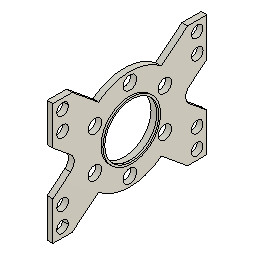
Ru28_Connector (Autodesk Fusion 360 design; units mm, degrees)
Autodesk Fusion 360 part; units mm, degrees
sketch "Sketch1" plane through (0, 0, 0) normal (0, 0, 1) x (1, 0, 0) in component "FINALBASE__2.0 v63"
  line L0 (175, -25) -> (0, -25)
  line L1 (0, -25) -> (0, 25)
  line L2 (0, 25) -> (175, 25)
  line L3 (175, 25) -> (175, -25)
  constraint horizontal L0
  constraint vertical L1
  constraint horizontal L2
  constraint vertical L3
extrude "Extrude1" add sketch "Sketch1" along normal blind 5 makes body 1 in component "FINALBASE__2.0 v63"
sketch "Sketch2" plane through (175, 0, 0) normal (1, 0, 0) x (0, 1, 0) in component "FINALBASE__2.0 v63"
  circle A0 centre (-0.0248, 31.4535) radius 20.9965 construction
  circle A1 centre (-0.0248, 31.4535) radius 22.3327
  line L0 (25, 0) -> (-25.0497, 0)
  line L1 (-25.0497, 0) -> (-25.0497, 62.9071)
  line L2 (-25.0497, 62.9071) -> (25, 62.9071)
  line L3 (25, 62.9071) -> (25, 0)
  line L4 (25, 0) -> (-25.0497, 62.9071) construction
  line L5 (-25.0497, 0) -> (25, 62.9071) construction
  line L6 (-0.0248, 31.4535) -> (-25.0497, 31.4535)
  line L7 (-0.0248, 31.4535) -> (25, 31.4535)
  point P0 (-0.0248, 31.4535)
  constraint concentric A0 A1
  constraint horizontal L0
  constraint perpendicular L0 L1
  constraint parallel L0 L2
  constraint parallel L1 L3
  constraint coincident L4 P0
  constraint coincident L5 P0
  constraint coincident P0 A0.centre
  constraint midpoint L1 L6.end
  constraint midpoint L3 L7.end
extrude "Extrude2" add sketch "Sketch2" along normal blind -52 and the other way blind 14 contours A1 L0 L1 L3 L6 L7 bodies 1 in component "FINALBASE__2.0 v63"
extrude "Extrude3" add 1 faces at (123, 0.548, 6.3944) along direction (-1, 0, 0) blind 95 and the other way blind -42 on bodies 1 bodies 1 in component "FINALBASE__2.0 v63"
fillet "Fillet1" radius 5 2 edges at (81, 0, 5) (123, 0, 5) on bodies 1 in component "FINALBASE__2.0 v63"
sketch "Sketch3" plane through (0, 0, 31.4535) normal (0, 0, 1) x (-1, 0, 0) in component "FINALBASE__2.0 v63"
  line L0 (-161, -25) -> (-123, -25) construction
  line L1 (-123, -25) -> (-123, 25) construction
  line L2 (-123, 25) -> (-161, 25) construction
  line L3 (-161, 25) -> (-161, -25) construction
  line L4 (-81, -25) -> (-28, -25) construction
  line L5 (-28, -25) -> (-28, 25) construction
  line L6 (-28, 25) -> (-81, 25) construction
  line L7 (-81, 25) -> (-81, -25) construction
  line L8 (-161, 25) -> (-123, 25)
  line L9 (-123, 25) -> (-123, 40)
  line L10 (-123, 40) -> (-161, 40)
  line L11 (-161, 40) -> (-161, 25)
  line L12 (-161, -25) -> (-123, -25)
  line L13 (-123, -25) -> (-123, -40)
  line L14 (-123, -40) -> (-161, -40)
  line L15 (-161, -40) -> (-161, -25)
  line L16 (-81, 25) -> (-28, 25)
  line L17 (-28, 25) -> (-28, 40)
  line L18 (-28, 40) -> (-81, 40)
  line L19 (-81, 40) -> (-81, 25)
  line L20 (-81, -25) -> (-28, -25)
  line L21 (-28, -25) -> (-28, -40)
  line L22 (-28, -40) -> (-81, -40)
  line L23 (-81, -40) -> (-81, -25)
  constraint horizontal L0
  constraint vertical L1
  constraint horizontal L2
  constraint vertical L3
  constraint horizontal L4
  constraint vertical L5
  constraint horizontal L6
  constraint vertical L7
  constraint horizontal L8
  constraint vertical L9
  constraint horizontal L10
  constraint vertical L11
  constraint horizontal L12
  constraint vertical L13
  constraint horizontal L14
  constraint vertical L15
  constraint horizontal L16
  constraint vertical L17
  constraint horizontal L18
  constraint vertical L19
  constraint horizontal L20
  constraint vertical L21
  constraint horizontal L22
  constraint vertical L23
  constraint collinear L17 L21
extrude "Extrude4" add sketch "Sketch3" against normal blind 5 bodies 1 in component "FINALBASE__2.0 v63"
sketch "Sketch4" plane through (0, 0, 31.4535) normal (0, 0, 1) x (-1, 0, 0) in component "FINALBASE__2.0 v63"
  line L0 (-161.054, -40.0324) -> (-28.0724, -40.0324) construction
  line L1 (-28.0724, -40.0324) -> (-28.0724, 39.9564) construction
  line L2 (-28.0724, 39.9564) -> (-161.054, 39.9564) construction
  line L3 (-161.054, 39.9564) -> (-161.054, -40.0324) construction
  circle A0 centre (-94.5861, 0) radius 77.5924 construction
  line L4 (-155.2801, 34.0099) -> (-33.892, 34.0099) construction
  line L5 (-33.892, 34.0099) -> (-33.892, -34.0099) construction
  line L6 (-33.892, -34.0099) -> (-155.2801, -34.0099) construction
  line L7 (-155.2801, -34.0099) -> (-155.2801, 34.0099) construction
  line L8 (-155.2801, 34.0099) -> (-33.892, -34.0099) construction
  line L9 (-33.892, 34.0099) -> (-155.2801, -34.0099) construction
  line L10 (-145.5079, 34.0099) -> (-43.6642, 34.0099) construction
  line L11 (-43.6642, 34.0099) -> (-43.6642, -34.0099) construction
  line L12 (-43.6642, -34.0099) -> (-145.5079, -34.0099) construction
  line L13 (-145.5079, -34.0099) -> (-145.5079, 34.0099) construction
  line L14 (-145.5079, 34.0099) -> (-43.6642, -34.0099) construction
  line L15 (-43.6642, 34.0099) -> (-145.5079, -34.0099) construction
  line L16 (-133.9419, 34.0099) -> (-55.2302, 34.0099) construction
  line L17 (-55.2302, 34.0099) -> (-55.2302, -34.0099) construction
  line L18 (-55.2302, -34.0099) -> (-133.9419, -34.0099) construction
  line L19 (-133.9419, -34.0099) -> (-133.9419, 34.0099) construction
  line L20 (-133.9419, 34.0099) -> (-55.2302, -34.0099) construction
  line L21 (-55.2302, 34.0099) -> (-133.9419, -34.0099) construction
  circle A1 centre (-155.2801, 34.0099) radius 2.5
  circle A2 centre (-145.5079, 34.0099) radius 2.5
  circle A3 centre (-133.9419, 34.0099) radius 2.5
  circle A4 centre (-55.2302, 34.0099) radius 2.5
  circle A5 centre (-43.6642, 34.0099) radius 2.5
  line L22 (-94.5861, 0) -> (-172.1785, 0) construction
  line L23 (-133.9419, -34.0099) -> (-55.2302, -34.0099) construction
  circle A6 centre (-155.2801, -34.0099) radius 2.5
  circle A7 centre (-133.9419, -34.0099) radius 2.5
  line L24 (-155.2801, -34.0099) -> (-33.892, -34.0099) construction
  circle A8 centre (-55.2302, -34.0099) radius 2.5
  circle A9 centre (-43.6642, -34.0099) radius 2.5
  circle A10 centre (-145.5079, -34.0099) radius 2.5
  line L25 (-145.5079, -34.0099) -> (-43.6642, -34.0099) construction
  circle A11 centre (-74.2255, 34.0099) radius 2.5
  circle A12 centre (-74.2255, -34.0099) radius 2.5
  point P0 (-94.5861, 0)
  point P1 (-94.5861, 0)
  point P2 (-94.5861, 0)
  constraint horizontal L0
  constraint vertical L1
  constraint horizontal L2
  constraint vertical L3
  constraint coincident L1.end A0
  constraint coincident L0.start A0
  constraint horizontal L4
  constraint perpendicular L4 L5
  constraint parallel L4 L6
  constraint parallel L5 L7
  constraint coincident L8 P2
  constraint coincident L9 P2
  constraint coincident P2 P1
  constraint horizontal L10
  constraint perpendicular L10 L11
  constraint parallel L10 L12
  constraint parallel L11 L13
  constraint coincident L14 P2
  constraint coincident L15 P2
  constraint coincident L4 L10.start
  constraint horizontal L16
  constraint perpendicular L16 L17
  constraint parallel L16 L18
  constraint parallel L17 L19
  constraint coincident L20 P2
  constraint coincident L21 P2
  constraint coincident L4 L16.start
  constraint coincident L4.start L7.end
  constraint coincident L10.start L13.end
  constraint coincident L16.start L19.end
  constraint coincident L16.end L17.start
  constraint coincident L10.end L11.start
  constraint coincident A0 L22.end
  constraint perpendicular L3 L22
  constraint symmetric L4.start L22 L6.end
  constraint symmetric L4.end L22 L5.end
  constraint symmetric L10.start L22 L12.end
  constraint symmetric L10.end L22 L11.end
  constraint symmetric L16.start L22 L18.end
  constraint symmetric L16.end L22 L17.end
  constraint symmetric A1 L22 A6
  constraint symmetric A2 L22 A10
  constraint symmetric A3 L22 A7
  constraint symmetric A4 L22 A8
  constraint symmetric A5 L22 A9
  constraint coincident L4 A11.centre
  constraint coincident L25 A12.centre
extrude "Extrude5" cut sketch "Sketch4" against normal blind 25 bodies 1 in component "FINALBASE__2.0 v63"
sketch "Sketch5" plane through (28, 0, 0) normal (-1, 0, 0) x (0, -1, 0) in component "FINALBASE__2.0 v63"
  circle A0 centre (0.0017, 31.4517) radius 25.9983
  circle A1 centre (0.0017, 31.4517) radius 5.6
  line L0 (0.0017, 31.4517) -> (0.0017, 39.4517) construction
  line L1 (0.0017, 31.4517) -> (0.0017, 52.4517) construction
  circle A2 centre (0.0017, 39.4517) radius 1.75
  circle A3 centre (0.0017, 52.4517) radius 3.5
  circle A4 centre (-18.1848, 41.9517) radius 3.5
  circle A5 centre (-18.1848, 20.9517) radius 3.5
  circle A6 centre (0.0017, 10.4517) radius 3.5
  circle A7 centre (18.1883, 20.9517) radius 3.5
  circle A8 centre (18.1883, 41.9517) radius 3.5
  circle A9 centre (-7.9983, 31.4517) radius 1.75
  circle A10 centre (0.0017, 23.4517) radius 1.75
  circle A11 centre (8.0017, 31.4517) radius 1.75
  circle A12 centre (0.0017, 31.4517) radius 14
  dimension "d37" = 360
  dimension "d39" = 360
  constraint concentric A0 A1
  constraint coincident A0.centre A1.centre
  constraint vertical L0
  constraint parallel L0 L1
  constraint coincident L0.end A2.centre
  constraint coincident L1.end A3.centre
  constraint concentric A1 A12
extrude "Extrude6" add sketch "Sketch5" along normal blind 9 and the other way blind -6 separate body contours A0 makes body 2 in component "FINALBASE__2.0 v63"
move_body "Move1" bodies 2 to x (1, 0, 0) y (0, 1, 0) z (0, 0, 1) at (1.2449, 0, 0) in component "FINALBASE__2.0 v63"
extrude "Extrude9" cut 1 faces at (18.6667, -8.3333, 5) along direction (0, 0, -1) blind 15 on bodies 1 bodies 1 in component "FINALBASE__2.0 v63"
copy_body "CopyPasteBodies2" bodies 1 makes body 3 in component "FINALBASE__2.0 v63"
move_body "Move2" bodies 3 to x (1, 0, 0) y (0, -1, 0) z (0, 0, -1) at (0, -7.6406, 70.0083) in component "FINALBASE__2.0 v63"
move_body "Move3" bodies 3 to x (1, 0, 0) y (0, 1, 0) z (0, 0, 1) at (0, 7.6406, -6.2174) in component "FINALBASE__2.0 v63"
extrude "Extrude10" add 6 faces at (28, 0.9221, 60.6964) (28, -30, 34.0041) (28, 30.0331, 35.6707) (28, -0.9221, 3.0945) (28, 30, 29.7869) (28, -30.0331, 29.7869) along direction (-1, 0, 0) blind 5 on bodies 1 3 bodies 3 1 in component "FINALBASE__2.0 v63"
move_body "Move4" bodies 2 to x (1, 0, 0) y (0, 1, 0) z (0, 0, 1) at (-1.0312, 0, 0) in component "FINALBASE__2.0 v63"
sketch "Sketch7" plane through (23, 0, 0) normal (-1, 0, 0) x (0, -1, 0) in component "FINALBASE__2.0 v63"
  line L0 (-24.9986, 62.907) -> (-40, 62.907)
  line L1 (-40, 62.907) -> (-40, 36)
  line L2 (-40, 36) -> (-24.6084, 36)
  line L3 (-24.6084, 36) -> (-24.9986, 62.907)
  line L4 (-40, 26.4538) -> (-25, 26.4538)
  line L5 (-25, 26.4538) -> (-25, 0)
  line L6 (-25, 0) -> (-40, 0)
  line L7 (-40, 0) -> (-40, 26.4538)
  line L8 (25, 0) -> (40.0001, 0)
  line L9 (40.0001, 0) -> (40.0001, 26.4538)
  line L10 (40.0001, 26.4538) -> (25, 26.4538)
  line L11 (25, 26.4538) -> (25, 0)
  line L12 (24.9999, 62.907) -> (40.0046, 62.907)
  line L13 (40.0046, 62.907) -> (40.0046, 36.3556)
  line L14 (40.0046, 36.3556) -> (24.9999, 36.3556)
  line L15 (24.9999, 36.3556) -> (24.9999, 62.907)
  constraint horizontal L0
  constraint perpendicular L0 L1
  constraint perpendicular L1 L2
  constraint horizontal L4
  constraint vertical L5
  constraint horizontal L6
  constraint vertical L7
  constraint horizontal L8
  constraint vertical L9
  constraint horizontal L10
  constraint vertical L11
  constraint horizontal L12
  constraint vertical L13
  constraint horizontal L14
  constraint vertical L15
extrude "Extrude11" add sketch "Sketch7" against normal blind 10 bodies 1 3 in component "FINALBASE__2.0 v63"
sketch "Sketch8" plane through (23, 0, 0) normal (-1, 0, 0) x (0, -1, 0) in component "FINALBASE__2.0 v63"
  line L0 (-39.9502, 31.4426) -> (40, 31.4426) construction
  line L1 (40, 31.4426) -> (40, 0) construction
  line L2 (40, 0) -> (-39.9502, 0) construction
  line L3 (-39.9502, 0) -> (-39.9502, 31.4426) construction
  circle A0 centre (0.0249, 15.7213) radius 42.9554 construction
  line L4 (35, 5) -> (-34.9502, 5) construction
  line L5 (-34.9502, 5) -> (-34.9502, 26.4426) construction
  line L6 (-34.9502, 26.4426) -> (35, 26.4426) construction
  line L7 (35, 26.4426) -> (35, 5) construction
  line L8 (35, 5) -> (-34.9502, 26.4426) construction
  line L9 (-34.9502, 5) -> (35, 26.4426) construction
  circle A1 centre (-34.9502, 5) radius 3
  circle A2 centre (35, 5) radius 3
  circle A3 centre (35, 15) radius 3
  circle A4 centre (-34.9502, 15) radius 3
  point P0 (0.0249, 15.7213)
  constraint horizontal L0
  constraint vertical L1
  constraint horizontal L2
  constraint vertical L3
  constraint coincident L1.end A0
  constraint coincident L0.start A0
  constraint horizontal L4
  constraint perpendicular L4 L5
  constraint parallel L4 L6
  constraint parallel L5 L7
  constraint coincident L8 P0
  constraint coincident L9 P0
  constraint coincident P0 A0.centre
  constraint coincident L4.end L5.start
  constraint coincident L4.start L7.end
  constraint coincident L7 A3.centre
  constraint coincident L5 A4.centre
fillet "Fillet4" radius 5 2 edges at (28, -40.0001, 0) (28, 40, 0) on bodies 1 in component "FINALBASE__2.0 v63"
extrude "Extrude12" cut sketch "Sketch8" against normal blind 19 bodies 1 in component "FINALBASE__2.0 v63"
sketch "Sketch9" plane through (19.2137, 0, 0) normal (-1, 0, 0) x (0, -1, 0) in component "FINALBASE__2.0 v63"
  circle A0 centre (-35, 15) radius 3
  circle A1 centre (-35, 5) radius 3
  circle A2 centre (35, 15) radius 3
  circle A3 centre (35, 5) radius 3
  line L0 (-40.0279, -0.0127) -> (-29.9908, -0.0127)
  line L1 (-29.9908, -0.0127) -> (-29.9908, 20.0387)
  line L2 (-29.9908, 20.0387) -> (-40.0279, 20.0387)
  line L3 (-40.0279, 20.0387) -> (-40.0279, -0.0127)
  line L4 (-40.0279, 20.0387) -> (-26, 31.5437)
  line L5 (-26, 31.5437) -> (-21.9991, 19.0005)
  line L6 (-21.9991, 19.0005) -> (-15.52, 11.8555)
  line L7 (-15.52, 11.8555) -> (-29.9908, -0.0127)
  circle A4 centre (-0.0152, 31.475) radius 14.025
  line L8 (-0.0152, 31.475) -> (0, 0) construction
  line L9 (0, 0) -> (-0.0152, 31.475) construction
  line L10 (-0.0152, 31.475) -> (-41.5149, 31.45) construction
  line L11 (40.0086, 20.0773) -> (25.9696, 31.5688)
  line L12 (25.9696, 31.5688) -> (21.9807, 19.0217)
  line L13 (21.9807, 19.0217) -> (15.5086, 11.8705)
  line L14 (15.5086, 11.8705) -> (29.9908, 0.0162)
  line L15 (29.9715, 20.0676) -> (40.0086, 20.0773)
  line L16 (29.9908, 0.0162) -> (29.9715, 20.0676)
  line L17 (40.0086, 20.0773) -> (40.0279, 0.0259)
  circle A5 centre (34.9952, 5.0338) radius 3
  line L18 (40.0279, 0.0259) -> (29.9908, 0.0162)
  line L19 (29.9529, 62.9699) -> (29.9577, 42.9185)
  circle A6 centre (34.9633, 57.9584) radius 3
  line L20 (-0.0152, 31.475) -> (-0.0379, 62.95) construction
  line L21 (-0.0379, 62.95) -> (-0.0152, 31.475) construction
  circle A7 centre (-35.0198, 47.9078) radius 3
  line L22 (39.99, 62.9723) -> (29.9529, 62.9699)
  line L23 (29.9577, 42.9185) -> (39.9948, 42.9209)
  line L24 (15.4849, 51.0982) -> (29.9529, 62.9699)
  circle A8 centre (34.9801, 47.9922) radius 3
  line L25 (39.9948, 42.9209) -> (25.9697, 31.4125)
  line L26 (-22.0141, 43.923) -> (-15.5436, 51.0758)
  circle A9 centre (34.9681, 57.9922) radius 3
  line L27 (-25.9999, 31.375) -> (-22.0141, 43.923)
  line L28 (39.9948, 42.9209) -> (39.99, 62.9723)
  line L29 (-40.0417, 42.8631) -> (-25.9999, 31.375)
  line L30 (25.9697, 31.4125) -> (21.9657, 43.9548)
  line L31 (-15.5436, 51.0758) -> (-30.0287, 62.9266)
  line L32 (-30.0046, 42.8752) -> (-40.0417, 42.8631)
  circle A10 centre (-35.0319, 57.9078) radius 3
  line L33 (-30.0287, 62.9266) -> (-30.0046, 42.8752)
  line L34 (-40.0658, 62.9145) -> (-30.0287, 62.9266)
  line L35 (21.9657, 43.9548) -> (15.4849, 51.0982)
  line L36 (-40.0417, 42.8631) -> (-40.0658, 62.9145)
  point P0 (-0.0379, 62.95)
  point P1 (-0.0152, 31.475)
  point P2 (-41.5149, 31.45)
  constraint horizontal L0
  constraint vertical L1
  constraint horizontal L2
  constraint vertical L3
  constraint parallel L4 L7
  constraint coincident P1 A4.centre
  constraint coincident L8.end L9.start
  constraint symmetric A1 L8 A5
  constraint symmetric L0.start L8 L17.end
  constraint symmetric L0.end L8 L14.end
  constraint symmetric L1.end L8 L15.start
  constraint symmetric L2.end L8 L11.start
  constraint symmetric L4.end L8 L11.end
  constraint symmetric L5.end L8 L12.end
  constraint symmetric L6.end L8 L13.end
  constraint symmetric L8.end L10 L20.end
  constraint symmetric A0 L10 A7
  constraint symmetric A1 L10 A10
  constraint symmetric A2 L10 A8
  constraint symmetric A3 L10 A9
  constraint symmetric L0.start L10 L34.start
  constraint symmetric L0.end L10 L31.end
  constraint symmetric L1.end L10 L32.start
  constraint symmetric L2.end L10 L29.start
  constraint symmetric L4.end L10 L27.start
  constraint symmetric L5.end L10 L26.start
  constraint symmetric L6.end L10 L26.end
  constraint symmetric P1 L10 A4.centre
  constraint symmetric L8.end L10 P0
  constraint symmetric P2 L10 L10.end
  constraint symmetric L10 L11.start L23.end
  constraint symmetric L10 L11.end L25.end
  constraint symmetric L10 L12.end L30.end
  constraint symmetric L10 L13.end L24.start
  constraint symmetric L10 L14.end L19.start
  constraint symmetric L10 L15.start L19.end
  constraint symmetric L10 L17.end L22.start
  constraint symmetric L10 A5 A6
extrude "Extrude13" add sketch "Sketch9" against normal up to surface (3 mm away) contours L0 L1 L2 L3 | L1 L2 L4 L5 L6 L7 L27 L29 | L4 L5 L26 L27 L29 L31 L32 L33 | L4 L5 L27 L29 | L32 L33 L34 L36 | L11 L12 L13 L14 L15 L16 L25 L30 | L15 L16 L17 L18 | L11 L12 L25 L30 | L11 L12 L19 L23 L24 L25 L30 L35 | L19 L22 L23 L28 bodies 2 in component "FINALBASE__2.0 v63"
fillet "Fillet6" radius 5 2 edges at (20.7137, 26.1029, 31.4593) (20.7137, -26.0649, 31.4907) on bodies 2 in component "FINALBASE__2.0 v63"
move_body "Move5" bodies 2 to x (1, 0, 0) y (0, 1, 0) z (0, 0, 1) at (-3.5582, 0, 0) in component "FINALBASE__2.0 v63"
move_body "Move6" bodies 2 to x (1, 0, 0) y (0, 1, 0) z (0, 0, 1) at (4.1805, 0, 0) in component "FINALBASE__2.0 v63"
move_body "Move7" bodies 2 to x (1, 0, 0) y (0, 1, 0) z (0, 0, 1) at (-3.0872, 0, 0) in component "FINALBASE__2.0 v63"
extrude "Extrude14" add 3 faces at (23, 0.889, 3.0945) (23, -30.0331, 28.1203) (23, 30, 28.1203) along direction (-1, 0, 0) blind 2 on bodies 1 bodies 1 in component "FINALBASE__2.0 v63"
sketch "Sketch10" plane through (21, 0, 0) normal (-1, 0, 0) x (0, -1, 0) in component "FINALBASE__2.0 v63"
  line L0 (21, 18) -> (-20.8581, 18)
  line L1 (-20.8581, 18) -> (-20.8581, -1.0056)
  line L2 (-20.8581, -1.0056) -> (21, -1.0056)
  line L3 (21, -1.0056) -> (21, 18)
  line L4 (21, 18) -> (-20.8581, -1.0056) construction
  line L5 (-20.8581, 18) -> (21, -1.0056) construction
  line L6 (-20.8581, 7.8568) -> (21, 8.4972)
  point P0 (0.0709, 8.4972)
  constraint horizontal L0
  constraint perpendicular L0 L1
  constraint parallel L0 L2
  constraint parallel L1 L3
  constraint coincident L4 P0
  constraint coincident L5 P0
  constraint coincident L1 L6.start
  constraint midpoint L3 L6.end
extrude "Extrude15" add sketch "Sketch10" against normal blind 3 contours L0 L1 L3 L6 bodies 1 in component "FINALBASE__2.0 v63"
sketch "Sketch11" plane through (0, 0, 0) normal (0, 0, -1) x (1, 0, 0) in component "FINALBASE__2.0 v63"
  circle A0 centre (157.8495, 12) radius 4.7405
  line L0 (157.8495, 16.7405) -> (122.7944, 16.7405)
  line L1 (157.8495, 7.2595) -> (122.7944, 7.2595)
  circle A1 centre (122.7944, 12) radius 4.7405
  line L2 (74.4624, 7.6731) -> (37.9403, 7.6731)
  line L3 (74.4624, 16.3269) -> (37.9403, 16.3269)
  circle A2 centre (37.9403, 12) radius 4.3269
  circle A3 centre (74.4624, 12) radius 4.3269
  line L4 (175, 0) -> (20, 0) construction
  circle A4 centre (74.4624, -12) radius 4.3269
  line L5 (157.8495, -16.7405) -> (122.7944, -16.7405)
  circle A5 centre (37.9403, -12) radius 4.3269
  line L6 (157.8495, -7.2595) -> (122.7944, -7.2595)
  line L7 (74.4624, -16.3269) -> (37.9403, -16.3269)
  line L8 (74.4624, -7.6731) -> (37.9403, -7.6731)
  circle A6 centre (122.7944, -12) radius 4.7405
  circle A7 centre (157.8495, -12) radius 4.7405
  circle A8 centre (100, 20) radius 2.5
  circle A9 centre (100, 9.2) radius 2.5
  line L9 (97.5, 20) -> (97.5, 9)
  line L10 (102.5, 20) -> (102.5, 9.2)
  line L11 (175, 0) -> (20, 0) construction
  line L12 (97.5, -20) -> (97.5, -9)
  circle A10 centre (100, -20) radius 2.5
  circle A11 centre (100, -9.2) radius 2.5
  line L13 (102.5, -20) -> (102.5, -9.2)
  constraint coincident A0 L0.start
  constraint tangent A0 L0
  constraint horizontal L0
  constraint coincident A0 L1.start
  constraint tangent A0 L1
  constraint horizontal L1
  constraint coincident L1.end A1
  constraint tangent L1 A1
  constraint coincident L0.end A1
  constraint coincident L3.start A3
  constraint tangent L3 A3
  constraint horizontal L3
  constraint coincident L2.start A3
  constraint tangent L2 A3
  constraint horizontal L2
  constraint coincident L2.end A2
  constraint tangent L2 A2
  constraint coincident L3.end A2
  constraint parallel L2 L4
  constraint symmetric A0 L4 A7
  constraint symmetric L0.start L4 L5.start
  constraint symmetric L0.end L4 L5.end
  constraint symmetric L1.start L4 L6.start
  constraint symmetric L1.end L4 L6.end
  constraint symmetric A1 L4 A6
  constraint symmetric L2.end L4 L8.end
  constraint symmetric L2.start L4 L8.start
  constraint symmetric L3.start L4 L7.start
  constraint symmetric L3.end L4 L7.end
  constraint symmetric A2 L4 A5
  constraint symmetric A3 L4 A4
  constraint coincident A8 L9.start
  constraint vertical L9
  constraint coincident A8 L10.start
  constraint coincident A9 L10.end
  constraint tangent A9 L10
  constraint parallel L9 L10
  constraint tangent A8 L9
  constraint tangent A8 L10
  constraint symmetric L4 A8 A10
  constraint symmetric L4 A9 A11
  constraint symmetric L4 L9.start L12.start
  constraint symmetric L4 L9.end L12.end
  constraint symmetric L4 L10.start L13.start
  constraint symmetric L4 L10.end L13.end
extrude "Extrude16" cut sketch "Sketch11" against normal blind 28 bodies 1 in component "FINALBASE__2.0 v63"
delete_body "RemoveBody1" bodies 3 in component "FINALBASE__2.0 v63"
sketch "Sketch12" plane through (19.7488, 0, 0) normal (1, 0, 0) x (0, 1, 0) in component "FINALBASE__2.0 v63"
  circle A0 centre (1.0363, 30.4153) radius 21.2888 construction
  circle A1 centre (-0.0004, 52.4546) radius 3.5 construction
  circle A2 centre (-0.021, 31.4399) radius 26.0101 construction
  circle A3 centre (-0.021, 31.4399) radius 15
  circle A4 centre (-0.021, 31.4399) radius 14.018
  constraint concentric A2 A3
  constraint concentric A2 A4
extrude "Extrude17" add sketch "Sketch12" along normal blind 1 bodies 2 in component "FINALBASE__2.0 v63"
extrude "Extrude18" add 1 faces at (24, -4.7817, 16.7584) along direction (1, 0, 0) blind 2.5 on bodies 1 bodies 1 in component "FINALBASE__2.0 v63"
ref_plane "WorkPlane1" through (0, -75, 0) normal (0, 1, 0) x (0, 0, 1) in component "FINALBASE__2.0 v63"
extrude "Extrude19" add 1 faces at (107.3333, -25, 1.6667) along direction (0, -1, 0) up to surface (0.0497 mm away) on bodies 1 bodies 1 in component "FINALBASE__2.0 v63"
fillet "Fillet7" radius 1.5 10 edges at (81, -25.0497, 18.2268) (82.4645, -25.0497, 6.4645) (102, -25.0497, 5) (121.5355, -25.0497, 6.4645) (123, -25.0497, 18.2268) (123, 25, 18.2268) (121.5355, 25, 6.4645) (102, 25, 5) (82.4645, 25, 6.4645) (81, 25, 18.2268) on bodies 1 in component "FINALBASE__2.0 v63"
fillet "Fillet8" radius 2 8 edges at (80.5607, -24.6103, 26.4535) (56.25, -25.0497, 26.4535) (142.75, -25.0497, 26.4535) (123.4393, -24.6103, 26.4535) (56.25, 25, 26.4535) (80.5607, 24.5607, 26.4535) (123.4393, 24.5607, 26.4535) (142.75, 25, 26.4535) on bodies 1 in component "FINALBASE__2.0 v63"
sketch "Sketch14" plane through (0, 0, 0) normal (0, 0, -1) x (1, 0, 0) in component "FINALBASE__2.0 v63"
  line L0 (169.0214, 29.5822) -> (30.9786, 29.5822) construction
  line L1 (30.9786, -29.355) -> (169.0214, -29.355) construction
  line L2 (169.0214, -29.355) -> (169.0214, 29.5822) construction
  line L3 (169.0214, 29.5822) -> (30.9786, -29.355) construction
  line L4 (30.9786, 29.5822) -> (169.0214, -29.355) construction
  line L5 (165, 35) -> (175, 35)
  line L6 (175, 35) -> (175, 25)
  line L7 (175, 25) -> (165, 25)
  line L8 (165, 25) -> (165, 35)
  line L9 (165, -35) -> (175, -35)
  line L10 (175, -35) -> (175, -25)
  line L11 (175, -25) -> (165, -25)
  line L12 (165, -25) -> (165, -35)
  line L13 (59.8553, 24.853) -> (70.0105, 24.853)
  line L14 (70.0105, 24.853) -> (70.0105, 35)
  line L15 (70.0105, 35) -> (59.8553, 35)
  line L16 (59.8553, 35) -> (59.8553, 24.853)
  line L17 (60.1179, -24.8833) -> (70.2338, -24.8833)
  line L18 (70.2338, -24.8833) -> (70.2338, -35.0497)
  line L19 (70.2338, -35.0497) -> (60.1179, -35.0497)
  line L20 (60.1179, -35.0497) -> (60.1179, -24.8833)
  point P0 (100, 0.1136)
  constraint horizontal L0
  constraint parallel L0 L1
  constraint coincident L3 P0
  constraint coincident L4 P0
  constraint horizontal L5
  constraint vertical L6
  constraint horizontal L7
  constraint vertical L8
  constraint horizontal L9
  constraint vertical L10
  constraint horizontal L11
  constraint vertical L12
  constraint horizontal L13
  constraint vertical L14
  constraint horizontal L15
  constraint vertical L16
  constraint horizontal L17
  constraint vertical L18
  constraint horizontal L19
  constraint vertical L20
extrude "Extrude20" add sketch "Sketch14" against normal up to surface (5 mm away) bodies 1 in component "FINALBASE__2.0 v63"
sketch "Sketch15" plane through (0, 0, 5) normal (0, 0, 1) x (-1, 0, 0) in component "FINALBASE__2.0 v63"
  line L0 (-170, -30) -> (-170, 30) construction
  line L1 (-170, 30) -> (-65, 30) construction
  line L2 (-65, 30) -> (-65, -30) construction
  line L3 (-65, -30) -> (-170, -30) construction
  circle A0 centre (-170, 30) radius 2.5
  circle A1 centre (-65, 30) radius 2.5
  circle A2 centre (-170, -30) radius 2.5
  circle A3 centre (-65, -30) radius 2.5
  constraint perpendicular L0 L1
  constraint parallel L0 L2
  constraint parallel L1 L3
  constraint vertical L0
  constraint coincident L0.end L1.start
  constraint coincident L1.end L2.start
  constraint coincident L0.start L3.end
  constraint coincident L2.end L3.start
extrude "Extrude21" cut sketch "Sketch15" along normal mid plane 22 bodies 1 in component "FINALBASE__2.0 v63"
fillet "Fillet10" radius 5 2 edges at (65.1758, 25, 5) (64.9329, -25.0497, 5) on bodies 1 in component "FINALBASE__2.0 v63"
fillet "Fillet11" radius 5 4 edges at (60.1179, 25, 5) (70.2338, 25, 5) (70.0105, -25.0497, 5) (59.8553, -25.0497, 5) on bodies 1 in component "FINALBASE__2.0 v63"
sketch "Sketch16" plane through (21, 0, 0) normal (-1, 0, 0) x (0, -1, 0) in component "FINALBASE__2.0 v63"
  circle A0 centre (-25, 10) radius 5
  circle A1 centre (25, 10) radius 5
  circle A2 centre (-10, 10) radius 5
  circle A3 centre (10, 10) radius 5
  line L0 (-25, 15) -> (-10, 15)
  line L1 (-10, 5) -> (-25, 5)
  line L2 (10, 15) -> (25, 15)
  line L3 (25, 5) -> (10, 5)
  constraint coincident A0 L0.start
  constraint coincident A2 L0.end
  constraint tangent A2 L0
  constraint horizontal L0
  constraint coincident A2 L1.start
  constraint coincident A0 L1.end
  constraint tangent A0 L1
  constraint parallel L0 L1
  constraint coincident A3 L2.start
  constraint coincident A1 L2.end
  constraint tangent A1 L2
  constraint coincident A1 L3.start
  constraint coincident A3 L3.end
  constraint tangent A3 L3
sketch "Sketch17" plane through (161, 0, 0) normal (1, 0, 0) x (0, 1, 0) in component "FINALBASE__2.0 v63"
  line L0 (-25.1344, 31.3854) -> (25, 31.3854)
  line L1 (25, 31.3854) -> (25, 5)
  line L2 (25, 5) -> (-25.1344, 5)
  line L3 (-25.1344, 5) -> (-25.1344, 31.3854)
  constraint horizontal L0
  constraint vertical L1
  constraint horizontal L2
  constraint vertical L3
sketch "Sketch19" plane through (21, 0, 0) normal (-1, 0, 0) x (0, -1, 0) in component "FINALBASE__2.0 v63"
  circle A0 centre (0, 31.4516) radius 25.9922 construction
  circle A1 centre (-18.1848, 20.9517) radius 3.5
  circle A2 centre (-18.1848, 20.9517) radius 6.25
  circle A3 centre (0.0007, 10.4532) radius 6.25
  circle A4 centre (18.1855, 20.953) radius 6.25
  circle A5 centre (18.1848, 41.9514) radius 6.25
  circle A6 centre (-0.0007, 52.45) radius 6.25
  circle A7 centre (-18.1855, 41.9501) radius 6.25
  dimension "d123" = 360
  constraint concentric A1 A2
extrude "Extrude23" cut sketch "Sketch19" against normal blind 94 contours A1 | A2 | A3 | A4 bodies 1 in component "FINALBASE__2.0 v63"
extrude "Extrude24" add 1 faces at (24.6667, 4.2248, 18) along direction (0, 0, 1) blind 7 on bodies 1 bodies 1 in component "FINALBASE__2.0 v63"
copy_body "Body->Comp1" bodies 2 removing the originals makes body 4 in component "PhysMat"
delete_body "RemoveBody7" bodies 1 in component "FINALBASE__2.0 v63"
component "FINALBASE__2.0 v63" placed x (1, 0, 0) y (0, 1, 0) z (0, 0, 1) at (0, 0, 0)
component "PhysMat" placed x (1, 0, 0) y (0, 1, 0) z (0, 0, 1) at (0, 0, 0) in component "FINALBASE__2.0 v63"
